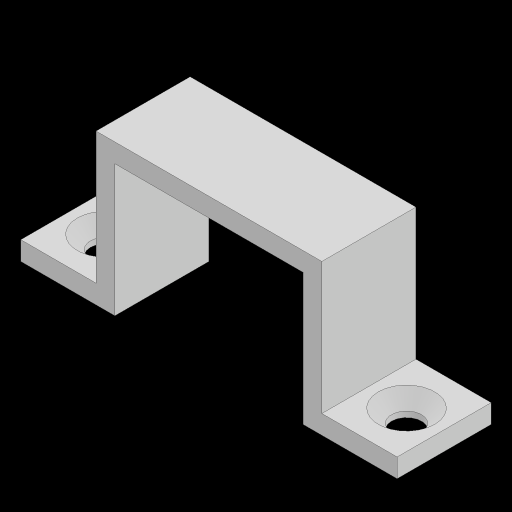
# Autodesk Inventor part: switchHolder
Saved by Autodesk Inventor 2024.3 (Build 283343010, 343A)
## iProperties
Created: 2025-04-30
Part Number: switchHolder
Material: Generic
Document SubType Name: Modeling
Designer: Oleg Kelner
Density: 1 g/cm^3
Appearance: Default
Author: Oleg Kelner
Autodesk Inventor part; units mm, degrees
ref_plane "YZ Plane" through (0, 0, 0) normal (1, 0, 0) x (0, 1, 0)
ref_plane "XZ Plane" through (0, 0, 0) normal (0, 1, 0) x (-1, 0, 0)
ref_plane "XY Plane" through (0, 0, 0) normal (0, 0, 1) x (1, 0, 0)
sketch "Sketch1" plane through (0, 0, 0) normal (0, 0, 1) x (1, 0, 0)
  line L0 (-10, 0) -> (10, 0) construction
  line L1 (10, 0) -> (10, 14)
  line L2 (10, 14) -> (-10, 14)
  line L3 (-10, 14) -> (-10, 0)
  line L4 (-12, -8.7582) -> (12, -8.7582) construction
  line L5 (12, -8.7582) -> (12, 2) construction
  line L6 (12, 16) -> (-12, 16)
  line L7 (-12, 16) -> (-12, 2)
  line L8 (-10, 0) -> (-20, 0)
  line L9 (-20, 0) -> (-20, 2)
  line L10 (-20, 2) -> (-12, 2)
  line L11 (-12, 2) -> (-12, -8.7582) construction
  line L12 (0, 16) -> (0, -8.7582)
  line L13 (10, 0) -> (20, 0)
  line L14 (20, 0) -> (20, 2)
  line L15 (20, 2) -> (12, 2)
  line L16 (12, 2) -> (12, 16)
  point P0 (0, 0)
  point P1 (0, 0)
  dimension "d0" = 14
  dimension "d1" = 20
  dimension "d2" = 2
  dimension "d3" = 2
  dimension "d4" = 10
  dimension "d5" = 2
  dimension "d6" = 2
  constraints: 34 end point, 7 parallel, 6 perpendicular, 3 midpoint, 3 symmetric about line, 2 horizontal, 1 coincident
  measures "d0" distance between parallel lines of L0 L2
  measures "d1" distance between parallel lines of L1 L3
  measures "d2" distance between parallel lines of L3 L7
  measures "d3" distance between parallel lines of L8 L10
  measures "d4" distance between parallel lines of L3 L9
  measures "d5" distance between parallel lines of L5 L1
  measures "d6" distance between parallel lines of L2 L6
extrude "Extrusion1" add sketch "Sketch1" along normal blind 10
sketch "Sketch2" plane through (-20, 2, 0) normal (0, 1, 0) x (1, 0, 0)
  line L0 (8, 0) -> (0, 0) construction
  line L1 (0, 0) -> (0, -10) construction
  line L2 (8, -10) -> (0, -10) construction
  line L3 (8, 0) -> (8, -10) construction
  line L4 (40, 0) -> (32, 0) construction
  line L5 (32, 0) -> (32, -10) construction
  line L6 (40, -10) -> (32, -10) construction
  line L7 (40, 0) -> (40, -10) construction
  line L8 (8, -10) -> (0, 0) construction
  line L9 (0, -10) -> (8, 0) construction
  line L10 (40, -10) -> (32, 0) construction
  line L11 (32, -10) -> (40, 0) construction
  point P0 (20, 0)
  point P1 (4, -5)
  point P2 (36, -5)
  constraints: 8 end point, 3 midpoint
hole "Hole1" at (-16, 2, 5) at (16, 2, 5) direction (0, -1, 0) diameter 3.2 end through all countersink diameter 6 countersink angle 90
body "Solid1"
